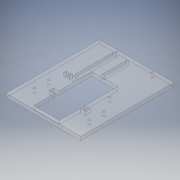
# Autodesk Inventor part: pibot_baseplate_battery
Saved by Autodesk Inventor 2018 (Build 220112000, 112)
## iProperties
Created: 2018-05-04
Part Number: pibot_baseplate_battery
Material: Polycarbonate, Clear
Document SubType Name: Sheet Metal
Designer: mmarkle
Density: 1.2 g/cm^3
Sheet Metal Rule: Default
Appearance: Polycarbonate - Clear
Author: mmarkle
Autodesk Inventor part; units mm, degrees
ref_plane "YZ Plane" through (0, 0, 0) normal (1, 0, 0) x (0, 1, 0)
ref_plane "XZ Plane" through (0, 0, 0) normal (0, 1, 0) x (-1, 0, 0)
ref_plane "XY Plane" through (0, 0, 0) normal (0, 0, 1) x (1, 0, 0)
sketch "Sketch1" plane through (0, 0, 0) normal (0, 1, 0) x (-1, 0, 0)
  line L0 (-50.8, 63.5) -> (50.8, 63.5)
  line L1 (50.8, 63.5) -> (50.8, -63.5)
  line L2 (50.8, -63.5) -> (-50.8, -63.5)
  line L3 (-50.8, -63.5) -> (-50.8, 63.5)
  line L4 (-50.8, 63.5) -> (50.8, -63.5) construction
  line L5 (50.8, 63.5) -> (-50.8, -63.5) construction
  point P0 (0, 0)
  point P1 (0, 0)
  dimension "d0" = 101.6
  dimension "d1" = 127
  measures "d0" distance of L1.end L2.end
  measures "d1" distance of L0.end L1.end
extrude "Plate1" add sketch "Sketch1" along normal blind 5.08
sketch "Sketch2" plane through (0, 5.08, 0) normal (0, 1, 0) x (1, 0, 0)
  line L0 (-50.8, 63.5) -> (50.8, 63.5) construction
  line L1 (0, 63.5) -> (0, -63.5) construction
  line L2 (50.8, -63.5) -> (-50.8, -63.5) construction
  line L3 (-50.8, -63.5) -> (-50.8, 63.5) construction
  point P0 (0, 0)
  point P1 (-37.338, -38.1)
  point P2 (-37.338, -18.542)
  point P3 (37.338, -38.1)
  point P4 (37.338, -18.542)
  dimension "d5" = 19.558
  dimension "d6" = 13.462
  dimension "d18" = 25.4
  constraints: 2 end point, 2 horizontal alignment, 2 midpoint, 2 vertical alignment, 1 symmetric about line
  measures "d5" distance of point (-37.338, -38.1) point (-37.338, -18.542)
  measures "d6" distance from line of L3 point (-37.338, -38.1)
  measures "d18" distance from line of point (-37.338, -38.1) L2
hole "MotorScrews" at (-37.338, 5.08, 38.1) at (-37.338, 5.08, 18.542) at (37.338, 5.08, 38.1) at (37.338, 5.08, 18.542) direction (0, -1, 0) diameter 3.2766 end through all clearance for "Flat Head Machine Screw (82)" size "#4" standard "Ansi Unified Screw Threads"
sketch "Sketch3" plane through (0, 5.08, 0) normal (0, 1, 0) x (1, 0, 0)
  line L0 (-17.5, -59.0917) -> (17.5, -59.0917)
  line L1 (17.5, -59.0917) -> (17.5, 20.2833)
  line L2 (17.5, 20.2833) -> (-17.5, 20.2833)
  line L3 (-17.5, 20.2833) -> (-17.5, -59.0917)
  line L4 (-17.5, -59.0917) -> (17.5, 20.2833) construction
  line L5 (17.5, -59.0917) -> (-17.5, 20.2833) construction
  point P0 (0, 0)
  point P1 (0, -19.4042)
  point P2 (0, -19.4042)
  dimension "d14" = 35
  dimension "d15" = 79.375
  constraints: 12 end point, 3 midpoint, 2 parallel, 1 horizontal, 1 perpendicular, 1 vertical alignment
  measures "d14" distance of L2.end L1.end
  measures "d15" distance of L1.end L0.end
extrude "BatteryHole" cut sketch "Sketch3" against normal blind 5.08
sketch "Sketch4" plane through (0, 5.08, 0) normal (0, 1, 0) x (1, 0, 0)
  line L0 (17.5, -59.0917) -> (-17.5, -59.0917) projected
  line L1 (-25.0073, -30.5582) -> (25.0073, -30.5582)
  line L2 (25.0073, -30.5582) -> (25.0073, -24.8469)
  line L3 (25.0073, -24.8469) -> (-25.0073, -24.8469)
  line L4 (-25.0073, -24.8469) -> (-25.0073, -30.5582)
  line L5 (-25.0073, -30.5582) -> (25.0073, -24.8469) construction
  line L6 (25.0073, -30.5582) -> (-25.0073, -24.8469) construction
  point P0 (0, 0)
  point P1 (0, -27.7026)
  point P2 (0, -27.7026)
  constraints: 12 end point, 2 midpoint, 2 parallel, 1 horizontal, 1 perpendicular, 1 vertical alignment
extrude "MotorWireHoles" cut sketch "Sketch4" against normal blind 5.08
sketch "Sketch5" plane through (0, 5.08, 0) normal (0, 1, 0) x (1, 0, 0)
  line L0 (0, 0) -> (0, 25.4) construction
  line L1 (-50.8, 63.5) -> (50.8, 63.5) projected
  point P0 (-24.4983, 2.3368)
  point P1 (24.4983, 2.3368)
  point P2 (-24.4983, 60.325)
  point P3 (24.4983, 60.325)
  dimension "d21" = 25.4
  dimension "d22" = 48.9966
  dimension "d23" = 57.9882
  dimension "d24" = 3.175
  constraints: 2 end point, 2 horizontal alignment, 2 vertical alignment, 1 symmetric about line, 1 vertical
  measures "d21" distance of L0.start L0.end
  measures "d22" distance of point (-24.498, 2.337) point (24.498, 2.337)
  measures "d23" distance of point (-24.498, 2.337) point (-24.498, 60.325)
  measures "d24" distance from line of L1 point (-24.498, 60.325)
hole "PiScrews" at (-24.4983, 5.08, -2.3368) at (24.4983, 5.08, -2.3368) at (-24.4983, 5.08, -60.325) at (24.4983, 5.08, -60.325) direction (0, -1, 0) diameter 2.8956 end through all clearance for "Flat Head Machine Screw" size "M2.5" standard "Ansi Metric M Profile"
sketch "Sketch6" plane through (0, 5.08, 0) normal (0, 1, 0) x (1, 0, 0)
  line L0 (-15.4305, 17.2899) -> (-15.4305, 42.6899) construction
  line L1 (-26.2255, 57.1039) -> (-23.0505, 57.1039)
  line L2 (-23.0505, 57.1039) -> (-23.0505, 6.3039)
  line L3 (-23.0505, 6.3039) -> (-26.2255, 6.3039)
  line L4 (-26.2255, 6.3039) -> (-26.2255, 57.1039)
  circle A0 centre (-24.4983, 60.325) radius 1.4478 projected
  line L5 (-4.6355, 57.1039) -> (-7.8105, 57.1039)
  line L6 (-7.8105, 57.1039) -> (-7.8105, 23.8538)
  line L7 (-7.8105, 23.8538) -> (-4.6355, 23.8538)
  line L8 (-4.6355, 23.8538) -> (-4.6355, 57.1039)
  dimension "d33" = 3.175
  dimension "d34" = 50.8
  dimension "d37" = 15.24
  constraints: 18 end point, 2 parallel, 2 symmetric about line, 1 horizontal, 1 perpendicular, 1 tangent, 1 vertical
  measures "d33" distance of L2.end L3.end
  measures "d34" distance of L1.end L2.end
  measures "d37" distance between parallel lines of L6 L2
extrude "WireHoles" cut sketch "Sketch6" against normal blind 5.08 contours L1 L2 L3 L4 | L8 L7 L6 L5
sketch "Sketch7" plane through (0, 5.08, 0) normal (0, 1, 0) x (1, 0, 0)
  line L0 (-36.0117, 4.0418) -> (-33.4717, 4.0418)
  line L1 (-33.4717, 4.0418) -> (-33.4717, 0.2318)
  line L2 (-33.4717, 0.2318) -> (-36.0117, 0.2318)
  line L3 (-36.0117, 0.2318) -> (-36.0117, 4.0418)
  line L4 (-30.3328, 4.1075) -> (-27.7928, 4.1075)
  line L5 (-27.7928, 4.1075) -> (-27.7928, 0.2975)
  line L6 (-27.7928, 0.2975) -> (-30.3328, 0.2975)
  line L7 (-30.3328, 0.2975) -> (-30.3328, 4.1075)
  point P0 (0, 0)
  dimension "d38" = 2.54
  dimension "d39" = 3.81
  dimension "d40" = 2.54
  dimension "d41" = 3.81
  constraints: 16 end point, 4 parallel, 2 horizontal, 2 perpendicular
  measures "d38" distance of L1.end L2.end
  measures "d39" distance of L0.end L1.end
  measures "d40" distance of L5.end L6.end
  measures "d41" distance of L4.end L5.end
extrude "ZipTieHolder" cut sketch "Sketch7" against normal blind 5.08
equation "\"d18\" = motor_placement"
equation "\"d12\" = Thickness"
equation "\"d16\" = Thickness"
equation "\"d19\" = Thickness"
equation "\"d30\" = Thickness"
equation "\"d35\" = Thickness"
equation "\"d42\" = Thickness"
equation "\"d4\" = Thickness"
equation "\"BendRadius\" = Thickness"
equation "\"BendReliefWidth\" = Thickness"
equation "\"BendReliefDepth\" = 0.5 * Thickness"
equation "\"CornerReliefSize\" = 4 * Thickness"
equation "\"MinimumRemnant\" = 2 * Thickness"
equation "\"TransitionRadius\" = BendRadius"
equation "\"JacobiRadiusSize\" = BendRadius"
equation "\"GapSize\" = Thickness"
equation "\"Thickness\" = 5.08"
equation "\"motor_placement\" = 25.4"
body "Solid1"
